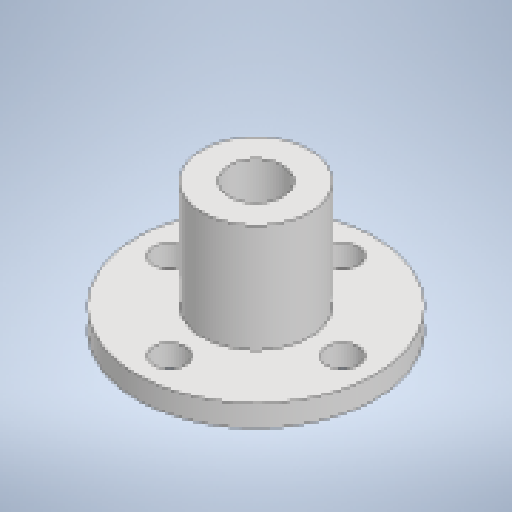
# Autodesk Inventor part: 5mm axle hub
Saved by Autodesk Inventor 2025 (Build 290162000, 162)
## iProperties
Created: 2025-08-04
Part Number: 5mm axle hub
Material: 一般
Document SubType Name: Modeling
Designer: gavin
Density: 1 g/cm^3
Appearance: 預設
Author: gavin
Autodesk Inventor part; units mm, degrees
ref_plane "YZ Plane" through (0, 0, 0) normal (1, 0, 0) x (0, 1, 0)
ref_plane "XZ Plane" through (0, 0, 0) normal (0, 1, 0) x (-1, 0, 0)
ref_plane "XY Plane" through (0, 0, 0) normal (0, 0, 1) x (1, 0, 0)
sketch "草圖1" plane through (0, 0, 0) normal (0, 1, 0) x (-1, 0, 0)
  circle A0 centre (0, 0) radius 11
  circle A1 centre (0, 0) radius 8 construction
  circle A2 centre (8, 0) radius 1.5
  circle A3 centre (0, 8) radius 1.5
  circle A4 centre (-8, 0) radius 1.5
  circle A5 centre (0, -8) radius 1.5
  dimension "d1" = 16
  dimension "d0" = 22
  dimension "d2" = 3
  dimension "d5" = 360
  constraints: 5 centre point, 2 coincident, 1 horizontal alignment, 11 other
  measures "d0" diameter of A0
  measures "d2" diameter of A2
extrude "擠出1" add sketch "草圖1" along normal blind 2
sketch "草圖2" plane through (0, 2, 0) normal (0, 1, 0) x (1, 0, 0)
  circle A0 centre (0, 0) radius 5
  dimension "d9" = 10
  constraints: 1 centre point, 1 coincident
  measures "d9" diameter of A0
extrude "擠出2" add sketch "草圖2" along normal blind 10
sketch "草圖3" plane through (0, 12, 0) normal (0, 1, 0) x (1, 0, 0)
  circle A0 centre (0, 0) radius 2.5
  dimension "d12" = 5
  constraints: 1 centre point, 1 coincident
  measures "d12" diameter of A0
extrude "擠出3" cut sketch "草圖3" against normal through all
